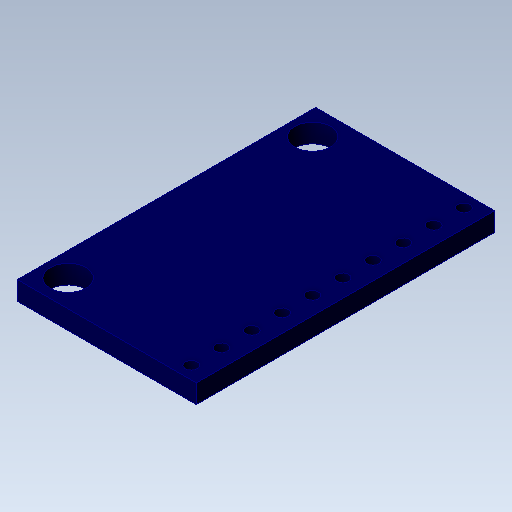
# Autodesk Inventor part: board
Saved by Autodesk Inventor 2020.3 (Build 243373000, 373)
## iProperties
Created: 2019-04-14
Part Number: board
Material: Generic
Document SubType Name: Modeling
Designer: ZEUSLAP
Density: 1 g/cm^3
Appearance: Default
Author: ZEUSLAP
Autodesk Inventor part; units mm, degrees
ref_plane "YZ Plane" through (0, 0, 0) normal (1, 0, 0) x (0, 1, 0)
ref_plane "XZ Plane" through (0, 0, 0) normal (0, 1, 0) x (-1, 0, 0)
ref_plane "XY Plane" through (0, 0, 0) normal (0, 0, 1) x (1, 0, 0)
sketch "Sketch1" plane through (0, 0, 0) normal (0, 1, 0) x (-1, 0, 0)
  line L0 (7.5, -12.5) -> (-7.5, -12.5)
  line L1 (-7.5, -12.5) -> (-7.5, 12.5)
  line L2 (-7.5, 12.5) -> (7.5, 12.5)
  line L3 (7.5, 12.5) -> (7.5, -12.5)
  line L4 (7.5, -12.5) -> (-7.5, 12.5) construction
  line L5 (-7.5, -12.5) -> (7.5, 12.5) construction
  circle A0 centre (5.5, 10.25) radius 1.5
  circle A1 centre (5.5, -10.25) radius 1.5
  line L6 (-6, 12.5) -> (-6, -12.5) construction
  circle A2 centre (-6, 11.43) radius 0.5
  circle A3 centre (-6, 8.89) radius 0.5
  circle A4 centre (-6, 6.35) radius 0.5
  circle A5 centre (-6, 3.81) radius 0.5
  circle A6 centre (-6, 1.27) radius 0.5
  circle A7 centre (-6, -1.27) radius 0.5
  circle A8 centre (-6, -3.81) radius 0.5
  circle A9 centre (-6, -6.35) radius 0.5
  circle A10 centre (-6, -8.89) radius 0.5
  circle A11 centre (-6, -11.43) radius 0.5
  point P0 (0, 0)
  dimension "d0" = 15
  dimension "d1" = 25
  dimension "d2" = 3
  dimension "d3" = 2.25
  dimension "d4" = 3
  dimension "d5" = 20.5
  dimension "d6" = 2.25
  dimension "d7" = 2
  dimension "d8" = 2
  dimension "d11" = 1.5
  dimension "d12" = 1
  dimension "d13" = 1.07
  dimension "d16" = 2.54
  dimension "d21" = 1.07
  constraints: 14 end point, 12 centre point, 3 point on line, 2 midpoint, 2 parallel, 2 vertical, 1 horizontal, 1 perpendicular, 18 other
  measures "d0" distance of L1.end L2.end
  measures "d1" distance of L0.end L1.end
  measures "d2" diameter of A0
  measures "d3" distance from line of L2 A0.centre
  measures "d4" diameter of A1
  measures "d5" distance of A1.centre A0.centre
  measures "d6" distance from line of L0 A1.centre
  measures "d7" distance from line of L3 A0.centre
  measures "d8" distance from line of L3 A1.centre
  measures "d11" distance between parallel lines of L1 L6
  measures "d12" diameter of A2
  measures "d13" distance from line of L2 A2.centre
  measures "d16" distance of A2.centre A3.centre
  measures "d21" distance from line of L0 A11.centre
extrude "Extrusion2" add sketch "Sketch1" along normal blind 1.57
body "Solid2"
